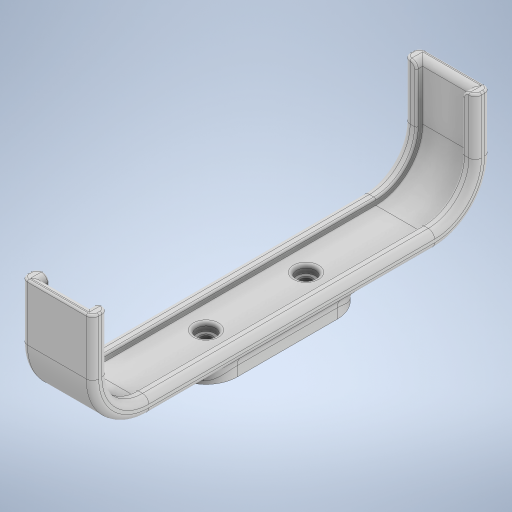
# Autodesk Inventor part: PlateGantryV2
Saved by Autodesk Inventor 2023 (Build 270158000, 158)
## iProperties
Created: 2026-01-22
Part Number: PlateGantryV2
Material: Generic
Document SubType Name: Modeling
Designer: DanAr
Density: 1 g/cm^3
Appearance: Default
Author: DanAr
Autodesk Inventor part; units mm, degrees
ref_plane "YZ Plane" through (0, 0, 0) normal (1, 0, 0) x (0, 1, 0)
ref_plane "XZ Plane" through (0, 0, 0) normal (0, 1, 0) x (-1, 0, 0)
ref_plane "XY Plane" through (0, 0, 0) normal (0, 0, 1) x (1, 0, 0)
sketch "Sketch1" plane through (0, 0, 0) normal (0, 1, 0) x (-1, 0, 0)
  line L0 (0, 0) -> (0, -32) construction
  line L1 (-10, 0) -> (-10, -32)
  line L2 (10, -32) -> (10, 0)
  arc A0 (10, 0) -> (-10, 0) centre (0, 0) ccw
  arc A1 (-10, -32) -> (10, -32) centre (0, -32) ccw
  circle A2 centre (0, 0) radius 1.7
  circle A3 centre (0, -32) radius 1.7
  point P0 (0, -16)
  dimension "d0" = 10
  dimension "d1" = 32
  dimension "d2" = 3.4
  constraints: 8 end point, 4 centre point, 4 point on circle, 4 tangent, 2 coincident, 1 midpoint, 1 parallel, 1 vertical
  measures "d0" radius of A1
  measures "d1" distance of L0.start L0.end
  measures "d2" diameter of A2
extrude "Extrusion1" add sketch "Sketch1" along normal blind 5
sketch "Sketch2" plane through (0, 5, 0) normal (0, 1, 0) x (1, 0, 0)
  circle A0 centre (0, 0) radius 1.7 projected
  circle A1 centre (0, 32) radius 1.7 projected
  line L0 (0, 0) -> (0, 32)
  line L1 (11.4, -48.7) -> (-11.4, -48.7)
  line L2 (-11.4, -48.7) -> (-11.4, 80.7)
  line L3 (-11.4, 80.7) -> (11.4, 80.7)
  line L4 (11.4, 80.7) -> (11.4, -48.7)
  line L5 (11.4, -48.7) -> (-11.4, 80.7) construction
  line L6 (-11.4, -48.7) -> (11.4, 80.7) construction
  circle A2 centre (0, 0) radius 1.7
  circle A3 centre (0, 32) radius 1.7
  point P0 (0, 16)
  dimension "d5" = 129.4
  dimension "d6" = 22.8
  constraints: 14 end point, 3 midpoint, 2 centre point, 2 coincident, 2 concentric, 2 parallel, 1 horizontal, 1 perpendicular
  measures "d5" distance of L1.end L2.end
  measures "d6" distance of L2.end L3.end
extrude "Extrusion2" add sketch "Sketch2" along normal blind 3
sketch "Sketch3" plane through (0, 8, 0) normal (0, 1, 0) x (1, 0, 0)
  line L0 (-11.4, 80.7) -> (-11.4, -48.7) projected
  line L1 (11.4, -48.7) -> (11.4, 80.7) projected
  line L2 (-11.4, -48.7) -> (11.4, -48.7)
  line L3 (11.4, -48.7) -> (11.4, -44.7)
  line L4 (11.4, -44.7) -> (-11.4, -44.7)
  line L5 (-11.4, -44.7) -> (-11.4, -48.7)
  line L6 (-11.4, 80.7) -> (11.4, 80.7)
  line L7 (11.4, 80.7) -> (11.4, 76.7)
  line L8 (11.4, 76.7) -> (-11.4, 76.7)
  line L9 (-11.4, 76.7) -> (-11.4, 80.7)
  line L10 (-11.4, -44.7) -> (-7.4, -44.7)
  line L11 (-7.4, -44.7) -> (-7.4, -40.7)
  line L12 (-7.4, -40.7) -> (-11.4, -40.7)
  line L13 (-11.4, -40.7) -> (-11.4, -44.7)
  line L14 (11.4, -44.7) -> (7.4, -44.7)
  line L15 (7.4, -44.7) -> (7.4, -40.7)
  line L16 (7.4, -40.7) -> (11.4, -40.7)
  line L17 (11.4, -40.7) -> (11.4, -44.7)
  line L18 (-11.4, 76.7) -> (-7.4, 76.7)
  line L19 (-7.4, 76.7) -> (-7.4, 72.7)
  line L20 (-7.4, 72.7) -> (-11.4, 72.7)
  line L21 (-11.4, 72.7) -> (-11.4, 76.7)
  line L22 (11.4, 76.7) -> (7.4, 76.7)
  line L23 (7.4, 76.7) -> (7.4, 72.7)
  line L24 (7.4, 72.7) -> (11.4, 72.7)
  line L25 (11.4, 72.7) -> (11.4, 76.7)
  point P0 (0, 0)
  dimension "d9" = 4
  dimension "d10" = 4
  dimension "d11" = 4
  dimension "d12" = 4
  dimension "d13" = 4
  dimension "d14" = 4
  dimension "d15" = 4
  dimension "d16" = 4
  dimension "d17" = 4
  dimension "d18" = 4
  constraints: 48 end point, 12 parallel, 6 horizontal, 6 perpendicular, 2 point on line
  measures "d9" distance between parallel lines of L2 L4
  measures "d10" distance between parallel lines of L6 L8
  measures "d11" distance of L11.end L12.end
  measures "d12" distance of L10.end L11.end
  measures "d13" distance of L14.end L15.end
  measures "d14" distance of L15.end L16.end
  measures "d15" distance of L19.end L20.end
  measures "d16" distance of L18.end L19.end
  measures "d17" distance of L22.end L23.end
  measures "d18" distance of L23.end L24.end
extrude "Extrusion3" add sketch "Sketch3" along normal blind 33 contours L6 L1 L8 L0 | L8 L19 L20 L0 | L1 L24 L23 L8 | L12 L11 L4 L0 | L4 L1 L2 L0 | L1 L4 L15 L16
sketch "Sketch4" plane through (0, 8, 0) normal (0, 1, 0) x (1, 0, 0)
  line L0 (-7.4, 72.7) -> (-11.4, 72.7) projected
  line L1 (7.4, -40.7) -> (11.4, -40.7) projected
  line L2 (-11.4, 72.7) -> (11.4, 72.7)
  line L3 (11.4, 72.7) -> (11.4, -40.7)
  line L4 (11.4, -40.7) -> (-11.4, -40.7)
  line L5 (-11.4, -40.7) -> (-11.4, 72.7)
  line L6 (7.4, -40.7) -> (7.4, -44.7) projected
  line L7 (-7.4, 76.7) -> (-7.4, 72.7) projected
  line L8 (7.4, -40.7) -> (-7.4, -40.7)
  line L9 (-7.4, -40.7) -> (-7.4, 72.7)
  line L10 (-7.4, 72.7) -> (7.4, 72.7)
  line L11 (7.4, 72.7) -> (7.4, -40.7)
  line L12 (7.4, -44.7) -> (-7.4, -44.7) projected
  line L13 (-7.4, 76.7) -> (7.4, 76.7) projected
  point P0 (0, 0)
  point P1 (7.4, 72.7)
  point P2 (-7.4, -40.7)
  dimension "d21" = 14.8
  dimension "d22" = 121.4
  constraints: 16 end point, 4 parallel, 2 horizontal, 2 perpendicular
  measures "d21" distance between parallel lines of L11 L9
  measures "d22" distance between parallel lines of L12 L13
extrude "Extrusion4" add sketch "Sketch4" along normal blind 4 contours L9 L4 L5 L0 | L2 L3 L1 L11
sketch "Sketch5" plane through (11.4, 5, 48.7) normal (1, 0, 0) x (0, 0, -1)
  line L0 (8, 7) -> (8, 36) projected
  line L1 (8, 36) -> (6, 36)
  line L2 (6, 36) -> (6, 7)
  line L3 (6, 7) -> (8, 7)
  line L4 (8, 7) -> (8, 36)
  line L5 (121.4, 7) -> (121.4, 36) projected
  line L6 (121.4, 36) -> (123.4, 36)
  line L7 (123.4, 36) -> (123.4, 7.21)
  line L8 (123.4, 7.21) -> (121.4, 7.21)
  line L9 (121.4, 7.21) -> (121.4, 36)
  line L10 (123.4, 7.21) -> (6, 7.21)
  line L11 (6, 7.21) -> (6, 5)
  line L12 (6, 5) -> (123.4, 5)
  line L13 (123.4, 5) -> (123.4, 7.21)
  point P0 (48.7, -5)
  point P1 (121.4, 7.21)
  point P2 (8, 7.21)
  dimension "d25" = 29
  dimension "d26" = 2
  dimension "d27" = 2
  dimension "d29" = 31
  constraints: 24 end point, 6 parallel, 3 horizontal, 3 perpendicular
  measures "d25" distance of L1.end L2.end
  measures "d26" distance of L2.end L3.end
  measures "d27" distance of L7.end L8.end
  measures "d29" distance between parallel lines of L1 L12
extrude "Extrusion5" cut sketch "Sketch5" against normal blind 60
sketch "Sketch6" plane through (11.4, 5, 48.7) normal (1, 0, 0) x (0, 0, -1)
  line L0 (0, 0) -> (0, 36) projected
  line L1 (129.4, 0) -> (0, 0) projected
  line L2 (0, 36) -> (1, 36)
  line L3 (1, 36) -> (1, 0)
  line L4 (1, 0) -> (0, 0)
  line L5 (0, 0) -> (0, 36)
  line L6 (129.4, 0) -> (129.4, 36) projected
  line L7 (129.4, 36) -> (128.4, 36)
  line L8 (128.4, 36) -> (128.4, 0)
  line L9 (128.4, 0) -> (129.4, 0)
  line L10 (129.4, 0) -> (129.4, 36)
  point P0 (48.7, -5)
  dimension "d32" = 1
  dimension "d33" = 1
  constraints: 16 end point, 4 parallel, 2 horizontal, 2 perpendicular, 2 point on line
  measures "d32" distance between parallel lines of L0 L3
  measures "d33" distance between parallel lines of L6 L8
extrude "Extrusion6" cut sketch "Sketch6" against normal blind 60
fillet "Fillet1" radius 13 4 edges at (-9.4, 10, -74.7) (9.4, 10, -74.7) (-9.4, 10, 42.7) (9.4, 10, 42.7)
fillet "Fillet2" radius 15 2 edges at (0, 8, -76.7) (0, 8, 44.7)
fillet "Fillet3" radius 18 2 edges at (0, 5, 47.7) (0, 5, -79.7)
sketch "Sketch7" plane through (0, 8, 0) normal (0, 1, 0) x (1, 0, 0)
  circle A0 centre (0, 32) radius 1.7 projected
  circle A1 centre (0, 32) radius 3
  circle A2 centre (0, 0) radius 1.7 projected
  circle A3 centre (0, 0) radius 3
  dimension "d39" = 6
  constraints: 2 centre point, 2 coincident
  measures "d39" diameter of A1
extrude "Extrusion7" cut sketch "Sketch7" against normal blind 2.5 contours A0 | A1 | A2 | A3
fillet "Fillet4" radius 2 10 edges at (11.4, 10.2721, -74.4279) (11.4, 32, -79.7) (11.4, 10.2721, 42.4279) (11.4, 32, 47.7) (11.4, 5, -16) (-11.4, 10.2721, -74.4279) (-11.4, 5, -16) (-11.4, 10.2721, 42.4279) (-11.4, 32, 47.7) (-11.4, 32, -79.7)
fillet "Fillet5" radius 4 16 edges at (10, 5.0921, -16) (9.8504, 5.0514, -33.723) (10, 5.0461, -32) (9.8489, 5, -33.7321) (0, 5, -42) (-9.8489, 5, -33.7321) (-9.8504, 5.0514, -33.723) (-10, 5.0461, -32) (-10, 5.0921, -16) (-9.8504, 5.0514, 1.723) (-9.8489, 5, 1.7321) (-10, 5.0461, 0) (9.8489, 5, 1.7321) (0, 5, 10) (9.8504, 5.0514, 1.723) (10, 5.0461, 0)
fillet "Fillet7" radius 2 6 edges at (7.4, 41, -75.7) (-7.4, 41, -75.7) (0, 41, -76.7) (-7.4, 41, 43.7) (7.4, 41, 43.7) (0, 41, 44.7)
fillet "Fillet8" radius 2 10 edges at (11.4, 32, -74.7) (11.4, 13.8076, -70.8924) (11.4, 10, -16) (11.4, 13.8076, 38.8924) (11.4, 32, 42.7) (-11.4, 13.8076, -70.8924) (-11.4, 10, -16) (-11.4, 13.8076, 38.8924) (-11.4, 32, 42.7) (-11.4, 32, -74.7)
fillet "Fillet9" radius 0.6 27 edges at (-7.4, 31, -74.7) (-7.4, 13.8076, -70.8924) (-7.4, 10, -16) (-7.4, 13.8076, 38.8924) (-7.4, 31, 42.7) (-7.9858, 40.4142, 42.7) (-10.8142, 41, 43.2858) (-11.4, 41, 45.2) (-10.8142, 41, 47.1142) (0, 41, 47.7) (10.8142, 41, 47.1142) (11.4, 41, 45.2) (10.8142, 41, 43.2858) (7.9858, 40.4142, 42.7) (7.4, 31, 42.7) (7.4, 13.8076, 38.8924) (7.4, 10, -16) (7.4, 31, -74.7) (7.9858, 40.4142, -74.7) (10.8142, 41, -75.2858) (11.4, 41, -77.2) (10.8142, 41, -79.1142) (0, 41, -79.7) (-10.8142, 41, -79.1142) (-11.4, 41, -77.2) (-10.8142, 41, -75.2858) (-7.9858, 40.4142, -74.7)
fillet "Fillet10" radius 1 2 edges at (-3, 8, 0) (-3, 8, -32)
chamfer "Chamfer1" distance 0.3 angle 45 2 edges at (-1.7, 5.5, -32) (-1.7, 5.5, 0)
sketch "Sketch8" plane through (10, 0, 0) normal (1, 0, 0) x (0, 0, -1)
  arc A0 (-42.7, 23) -> (-29.7, 10) centre (-29.7, 23) ccw projected
  line L0 (-29.7, 23) -> (-44.7, 23)
  line L1 (-44.7, 23) -> (-44.7, 8)
  line L2 (-44.7, 8) -> (-29.7, 8)
  line L3 (-29.7, 8) -> (-29.7, 23)
  line L4 (-44.7, 8) -> (76.7, 8)
  line L5 (76.7, 8) -> (76.7, 129.4)
  line L6 (76.7, 129.4) -> (-44.7, 129.4)
  line L7 (-44.7, 129.4) -> (-44.7, 8)
  line L8 (0, 0) -> (32, 0) projected
  dimension "d52" = 121.4
  dimension "d53" = 121.4
  dimension "d54" = 15
  dimension "d55" = 8
  constraints: 16 end point, 4 parallel, 2 horizontal, 2 perpendicular
  measures "d52" distance of L5.end L6.end
  measures "d53" distance of L4.end L5.end
  measures "d54" distance of L2.end L0.start
  measures "d55" distance between parallel lines of L8 L4
body "Solid1"
